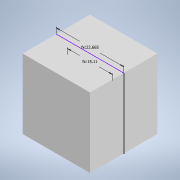
# Autodesk Inventor part: parametry
Saved by Autodesk Inventor 2022 (Build 260153000, 153)
## iProperties
Created: 2021-05-12
Part Number: parametry
Material: Všeobecné
Document SubType Name: Modeling
Designer: peepu
Density: 1 g/cm^3
Appearance: Výchozí
Author: peepu
Autodesk Inventor part; units mm, degrees
ref_plane "YZ Plane" through (0, 0, 0) normal (1, 0, 0) x (0, 1, 0)
ref_plane "XZ Plane" through (0, 0, 0) normal (0, 1, 0) x (-1, 0, 0)
ref_plane "XY Plane" through (0, 0, 0) normal (0, 0, 1) x (1, 0, 0)
sketch "Náčrt1" plane through (0, 0, 0) normal (0, 0, 1) x (1, 0, 0)
  circle A0 centre (0, 0) radius 7.5551
  line L0 (-7.5551, -7.5551) -> (7.5551, -7.5551)
  line L1 (7.5551, -7.5551) -> (7.5551, 7.5551)
  line L2 (7.5551, 7.5551) -> (-7.5551, 7.5551)
  line L3 (-7.5551, 7.5551) -> (-7.5551, -7.5551)
  line L4 (-7.5551, -7.5551) -> (7.5551, 7.5551) construction
  line L5 (7.5551, -7.5551) -> (-7.5551, 7.5551) construction
  line L6 (-11.3327, -11.713) -> (11.3327, -11.713)
  line L7 (11.3327, -11.713) -> (11.3327, 11.713)
  line L8 (11.3327, 11.713) -> (-11.3327, 11.713)
  line L9 (-11.3327, 11.713) -> (-11.3327, -11.713)
  line L10 (-11.3327, -11.713) -> (11.3327, 11.713) construction
  line L11 (11.3327, -11.713) -> (-11.3327, 11.713) construction
  line L12 (-7.5551, 0) -> (7.5551, 0)
  dimension "d1" = 15.1102
  dimension "d2" = 22.6653
  constraints: 26 end point, 6 midpoint, 4 parallel, 2 horizontal, 2 perpendicular, 1 centre point, 1 coincident
  measures "d1" distance of L2.end L1.end
  measures "d2" distance of L8.end L7.end
extrude "Vysunutí1" add sketch "Náčrt1" along normal mid plane 22.6653 contours L12 A0 | L1 L0 A0 | A0 L2 L1 | A0 L12 | A0 L3 L2 | L0 L3 A0 | L9 L8 L7 L6
extrude "Vysunutí2" cut sketch "Náčrt1" along normal mid plane 15.1102 contours L12 A0 | L1 L0 A0 | A0 L2 L1 | A0 L12 | A0 L3 L2 | L0 L3 A0
revolve "Rotace1" add sketch "Náčrt1" angle 360 about axis through (-7.5551, 0, 0) along (1, 0, 0) picked at (1.9689, 1.5702) contours L12 A0
equation "\"d1\" = PRUMER"
equation "\"d2\" = HRANA"
equation "\"d3\" = HRANA"
equation "\"d5\" = PRUMER"
equation "\"PRUMER\" = 15.11021"
equation "\"HRANA\" = 1.5 * PRUMER"
